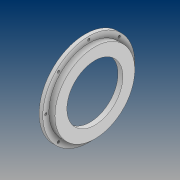
# Autodesk Inventor part: lavyrintosecondchance
Saved by Autodesk Inventor 2021 (Build 250183000, 183)
## iProperties
Created: 2021-01-08
Part Number: lavyrintosecondchance
Material: Generic
Document SubType Name: Modeling
Designer: Διογενης Τσιχλακης
Density: 1 g/cm^3
Appearance: Default
Author: Διογενης Τσιχλακης
Autodesk Inventor part; units mm, degrees
ref_plane "YZ Plane" through (0, 0, 0) normal (1, 0, 0) x (0, 1, 0)
ref_plane "XZ Plane" through (0, 0, 0) normal (0, 1, 0) x (-1, 0, 0)
ref_plane "XY Plane" through (0, 0, 0) normal (0, 0, 1) x (1, 0, 0)
sketch "Sketch1" plane through (0, 0, 0) normal (1, 0, 0) x (0, 1, 0)
  circle A0 centre (0, 0) radius 188.9
  circle A1 centre (0, 0) radius 163.9
  dimension "d0" = 377.8
  dimension "d2" = 327.8
  constraints: 2 centre point, 2 coincident
  measures "d0" diameter of A0
  measures "d2" diameter of A1
extrude "Extrusion1" add sketch "Sketch1" along normal blind 15
sketch "Sketch2" plane through (15, 0, 0) normal (1, 0, 0) x (0, 0, -1)
  circle A0 centre (0, 0) radius 176.5
  circle A1 centre (0, 176.5) radius 5
  dimension "d5" = 353
  dimension "d6" = 10
  constraints: 1 centre point, 1 coincident, 1 vertical alignment, 2 other
  measures "d6" diameter of A1
extrude "Extrusion2" cut sketch "Sketch2" against normal through all contours A1 A0 | A0 A1 picked at (0.1991, 174.84) picked at (0.1901, 178.1505)
pattern_circular "Circular Pattern1" count 8 over 360 about axis through (0, 0, 0) along (1, 0, 0) of "Extrusion2"
sketch "Sketch3" plane through (0, 0, 0) normal (-1, 0, 0) x (0, 0, 1)
  circle A0 centre (0, 0) radius 163.9
  circle A1 centre (0, 0) radius 158.9
  dimension "d12" = 317.8
  constraints: 2 centre point, 2 coincident
  measures "d12" diameter of A1
extrude "Extrusion3" add sketch "Sketch3" against normal blind 40
sketch "Sketch4" plane through (0, 0, 0) normal (0, 0, 1) x (1, 0, 0)
  line L0 (40, 158.9) -> (40, -158.9) projected
  line L1 (40, -163.9) -> (40, 163.9) projected
  line L2 (30, 153.9) -> (30, 158.9)
  line L3 (30, 158.9) -> (40, 158.9)
  line L4 (40, 158.9) -> (40, 153.9)
  line L5 (30, 153.9) -> (30, 134)
  line L6 (40, 134) -> (40, 153.9)
  line L7 (-8, 0) -> (48, 0) projected
  line L8 (40, 158.9) -> (40, 134)
  line L9 (30, 134) -> (20, 134)
  line L10 (20, 134) -> (20, 131)
  line L11 (20, 131) -> (30, 131)
  line L12 (30, 131) -> (30, 126)
  line L13 (30, 126) -> (20, 126)
  line L14 (20, 126) -> (20, 123)
  line L15 (20, 123) -> (30, 123)
  line L16 (30, 123) -> (30, 118)
  line L17 (30, 118) -> (20, 118)
  line L18 (20, 118) -> (20, 115)
  line L19 (20, 115) -> (40, 115)
  line L20 (40, 115) -> (40, 134)
  point P0 (0, 0)
  constraints: 36 end point, 10 perpendicular, 3 horizontal, 2 collinear, 2 point on line, 1 parallel, 1 vertical
revolve "Revolution1" add sketch "Sketch4" angle 360 about axis through (-10, 0, 0) along (1, 0, 0)
thread "Thread1" size "M10x1.5" class "6H" standard "ANSI Metric M Profile" full length
thread "Thread2" size "M10x1.5" class "6H" standard "ANSI Metric M Profile" full length
thread "Thread3" size "M10x1.5" class "6H" standard "ANSI Metric M Profile" full length
thread "Thread4" size "M10x1.5" class "6H" standard "ANSI Metric M Profile" full length
thread "Thread5" size "M10x1.5" class "6H" standard "ANSI Metric M Profile" full length
thread "Thread6" size "M10x1.5" class "6H" standard "ANSI Metric M Profile" full length
thread "Thread7" size "M10x1.5" class "6H" standard "ANSI Metric M Profile" full length
thread "Thread8" size "M10x1.5" class "6H" standard "ANSI Metric M Profile" full length
body "Solid1"
